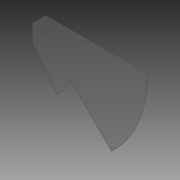
# Autodesk Inventor part: Shooter Top Shield
Saved by Autodesk Inventor 2014 SP1 (Build 180222100, 222)
## iProperties
Created: 2013-12-16
Part Number: Shooter Top Shield
Material: Polycarbonate, Clear
Document SubType Name: Modeling
Designer: Moses
Mass: 75.1588 g
Surface Area: 1588.6 cm^2
Volume: 62.6323 cm^3
Density: 1.2 g/cm^3
Appearance: Polycarbonate - Clear
Author: Moses
Autodesk Inventor part; units mm, degrees
ref_plane "YZ Plane" through (0, 0, 0) normal (1, 0, 0) x (0, 1, 0)
ref_plane "XZ Plane" through (0, 0, 0) normal (0, 1, 0) x (-1, 0, 0)
ref_plane "XY Plane" through (0, 0, 0) normal (0, 0, 1) x (1, 0, 0)
sketch "Sketch1" plane through (0, 0, 0) normal (0, 0, 1) x (1, 0, 0)
  circle A0 centre (-72.9692, 83.7456) radius 1.905 projected
  circle A1 centre (-6.9415, 6.9415) radius 3.3782 construction
  circle A2 centre (16.8562, -16.8562) radius 3.3782 construction
  circle A3 centre (38.5187, 116.692) radius 3.3782 construction
  circle A4 centre (-71.8903, 66.2616) radius 1.905 projected
  line L0 (12.4678, -30.4284) -> (152.5708, -170.5313) construction
  arc A5 (152.5708, -170.5313) -> (170.5313, -152.5708) centre (-116.692, 116.692) ccw construction
  line L1 (170.5313, -152.5708) -> (-82.3118, 100.2723) construction
  arc A6 (-82.3118, 100.2723) -> (-79.1249, 110.342) centre (-116.692, 116.692) ccw construction
  line L2 (-79.1249, 110.342) -> (276.9567, 110.342) construction
  arc A7 (276.9567, 110.342) -> (277.008, 116.692) centre (-116.692, 116.692) ccw construction
  line L3 (277.008, 116.692) -> (277.008, 123.042) construction
  line L4 (277.008, 123.042) -> (-79.1249, 123.042) construction
  arc A8 (-79.1249, 123.042) -> (-123.042, 79.1249) centre (-116.692, 116.692) ccw construction
  line L5 (-123.042, 79.1249) -> (-123.042, 17.0203) construction
  arc A9 (-110.342, 2.2518) -> (-123.042, 17.0203) centre (-227.182, -85.3782) ccw construction
  line L6 (-110.342, 2.2518) -> (-44.6195, -85.3782) construction
  line L7 (-44.6195, -85.3782) -> (-110.342, -173.0082) construction
  arc A10 (-123.042, -187.7768) -> (-110.342, -173.0082) centre (-227.182, -85.3782) ccw construction
  line L8 (-123.042, -187.7768) -> (-123.042, -277.008) construction
  line L9 (-123.042, -277.008) -> (-116.692, -277.008) construction
  arc A11 (-116.692, -277.008) -> (-110.342, -276.9567) centre (-116.692, 116.692) ccw construction
  line L10 (-110.342, -276.9567) -> (-110.342, -194.1749) construction
  line L11 (-110.342, -194.1749) -> (12.4678, -30.4284) construction
  circle A12 centre (-116.692, -270.658) radius 3.3782 construction
  circle A13 centre (-116.692, -219.858) radius 3.3782 construction
  line L12 (3.3964, -21.3569) -> (-36.682, -74.7949) construction
  line L13 (-36.682, -74.7949) -> (-110.342, 23.4184) construction
  line L14 (-110.342, 23.4184) -> (-110.342, 79.1249) construction
  arc A14 (-110.342, 79.1249) -> (-100.2723, 82.3118) centre (-116.692, 116.692) ccw construction
  line L15 (-100.2723, 82.3118) -> (3.3964, -21.3569) construction
  circle A15 centre (-116.692, 116.692) radius 9.5 construction
  circle A16 centre (153.5355, -160.8275) radius 3.3782 projected
  circle A17 centre (160.8275, -153.5355) radius 3.3782 construction
  circle A18 centre (117.6145, -124.9064) radius 3.3782 construction
  circle A19 centre (124.9064, -117.6145) radius 3.3782 construction
  circle A20 centre (270.658, 116.692) radius 3.3782 projected
  circle A21 centre (219.858, 116.692) radius 3.3782 construction
  circle A22 centre (23.008, 116.692) radius 3.3782 construction
  circle A23 centre (162.708, 116.692) radius 3.3782 construction
  circle A24 centre (-22.5015, 13.5212) radius 3.3782 construction
  circle A25 centre (-13.5212, 22.5015) radius 3.3782 construction
  circle A26 centre (76.3324, -85.3127) radius 3.3782 construction
  circle A27 centre (85.3127, -76.3324) radius 3.3782 construction
  line L16 (-79.1249, 123.042) -> (276.9567, 123.042)
  line L17 (-79.1249, 123.042) -> (-123.042, 79.1249)
  line L18 (-123.042, 79.1249) -> (-123.042, 17.0203)
  line L19 (-123.042, 17.0203) -> (-36.599, -95.8509)
  line L20 (-36.599, -95.8509) -> (12.4678, -30.4284)
  line L21 (12.4678, -30.4284) -> (152.5708, -170.5313)
  arc A28 (152.5708, -170.5313) -> (276.9567, 123.042) centre (-116.692, 116.692) ccw
  circle A29 centre (64.8391, -67.458) radius 1.7145 projected
  circle A30 centre (64.8391, 116.692) radius 1.7145 projected
  line L22 (72.3797, -92.858) -> (57.2985, -92.858) construction
  line L23 (72.3797, -92.858) -> (72.3797, 123.042) construction
  line L24 (57.2985, 123.042) -> (72.3797, 123.042) construction
  line L25 (57.2985, -92.858) -> (57.2985, 123.042) construction
  circle A31 centre (64.8391, 116.692) radius 1.7145 projected
  circle A32 centre (64.8391, -67.458) radius 1.7145 projected
  circle A33 centre (72.1737, 116.692) radius 3.3782 projected
  point P0 (0, 0)
  constraints: 12 end point, 3 point on line, 2 point on circle, 1 centre point, 1 coincident, 1 collinear, 1 parallel, 1 perpendicular
extrude "Extrusion1" add sketch "Sketch1" along normal blind 0.7937 contours L16 A28 L21 L20 L19 L18 L17 | A33
body "Solid1"
